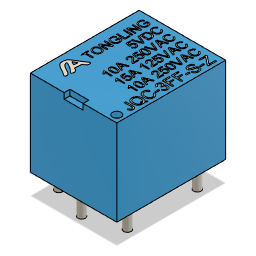
5v Cube Relay (Autodesk Fusion 360 design; units mm, degrees)
Autodesk Fusion 360 part; units mm, degrees
(part 1 of 2)
sketch "Sketch1" plane through (0, 0, 0) normal (0, 1, 0) x (1, 0, 0)
  line L0 (0, 0) -> (26, 0)
  line L1 (26, 0) -> (26, 33.5)
  line L2 (26, 33.5) -> (0, 33.5)
  line L3 (0, 33.5) -> (0, 0)
  line L4 (2.275, 33.5) -> (2.275, 0) construction
  circle A0 centre (2.275, 31.325) radius 1.475
  circle A1 centre (2.275, 2.375) radius 1.475
  line L5 (13, 33.5) -> (13, 0) construction
  circle A2 centre (23.725, 31.325) radius 1.475
  circle A3 centre (23.725, 2.375) radius 1.475
  dimension "d1" = 26
  dimension "d2" = 33.5
  dimension "d3" = 2.95
  dimension "d4" = 0.75
  dimension "d5" = 0.7
  dimension "d7" = 2.225
  dimension "d9" = 26
  dimension "d10" = 0.9
  dimension "d11" = 18.5
  constraint horizontal L0
  constraint vertical L1
  constraint horizontal L2
  constraint vertical L3
  constraint coincident L0.start L3.end
  constraint coincident L2 L4.start
  constraint coincident L0 L4.end
  constraint perpendicular L0 L4
  constraint coincident L4 A0.centre
  constraint coincident L4 A1.centre
  constraint equal A0 A1
  constraint midpoint L2 L5.start
  constraint midpoint L0 L5.end
  constraint symmetric A0 L5 A2
  constraint symmetric A1 L5 A3
  measures "d1" distance of L0.start L0.end
  measures "d2" distance of L0.start L2.end
  measures "d3" diameter of A0
  measures "d5" distance of L2 A0
  measures "d9" distance of A0 A1
  measures "d10" distance of L0 A1
  measures "d11" distance of A1 A3
sketch "Sketch2" plane through (0, 1.55, 0) normal (0, 1, 0) x (-1, 0, 0)
  circle A0 centre (-2.275, -2.375) radius 1.475
  circle A1 centre (-23.725, -2.375) radius 1.475
  circle A2 centre (-23.725, -31.325) radius 1.475
  circle A3 centre (-2.275, -31.325) radius 1.475
  line L0 (0, -33.5) -> (0, 0)
  line L1 (0, 0) -> (-26, 0)
  line L2 (-26, 0) -> (-26, -33.5)
  line L3 (-26, -33.5) -> (0, -33.5)
  line L4 (-5.9, -23.5) -> (-21, -23.5)
  line L5 (-21, -23.5) -> (-21, -4.5)
  line L6 (-21, -4.5) -> (-5.9, -4.5)
  line L7 (-5.9, -4.5) -> (-5.9, -23.5)
  dimension "d14" = 15.1
  dimension "d15" = 19
  dimension "d16" = 10
  dimension "d17" = 5
  dimension "d18" = 5.9
  dimension "d19" = 4.75
  constraint horizontal L4
  constraint vertical L5
  constraint horizontal L6
  constraint vertical L7
  measures "d14" distance of L4.start L4.end
  measures "d15" distance of L4.start L6.end
  measures "d16" distance of L3 L4
  measures "d17" distance of L2 L5
  measures "d18" distance of L0 L7
extrude "Extrude2" add sketch "Sketch2" along normal blind 15 contours L4 L5 L6 L7 makes body 1
sketch "Sketch3" plane through (0, 16.55, 0) normal (0, 1, 0) x (-1, 0, 0)
  line L0 (-5.9, -4.5) -> (-21, -4.5)
  line L1 (-21, -4.5) -> (-21, -23.5)
  line L2 (-21, -23.5) -> (-5.9, -23.5)
  line L3 (-5.9, -23.5) -> (-5.9, -4.5)
  circle A0 centre (-19.75, -5.75) radius 0.75
  line L4 (-15.1, -5.5) -> (-11.8, -5.5)
  line L5 (-11.8, -5.5) -> (-11.8, -3.5)
  line L6 (-11.8, -3.5) -> (-15.1, -3.5)
  line L7 (-15.1, -3.5) -> (-15.1, -5.5)
  line L8 (-15.1, -5.5) -> (-11.8, -3.5) construction
  line L9 (-11.8, -5.5) -> (-15.1, -3.5) construction
  point P0 (-13.45, -4.5)
  dimension "d22" = 1.5
  dimension "d23" = 0.5
  dimension "d24" = 0.5
  dimension "d25" = 1
  dimension "d26" = 3.3
  constraint horizontal L4
  constraint perpendicular L4 L5
  constraint parallel L4 L6
  constraint parallel L5 L7
  constraint coincident L8 P0
  constraint coincident L9 P0
  constraint midpoint L0 P0
  measures "d22" diameter of A0
  measures "d23" distance of L0 A0
  measures "d24" distance of L1 A0
  measures "d25" distance of L0 L4
  measures "d26" distance of L5.end L6.end
extrude "Extrude3" cut sketch "Sketch3" against normal blind 1 contours L0 L4 L5 L7 | L0 L5 L6 L7 | A0 bodies 1
sketch "Sketch4" plane through (0, 16.55, 0) normal (0, 1, 0) x (-1, 0, 0)
  line L0 (-11.8, -4.5) -> (-11.8, -5.5)
  line L1 (-11.8, -5.5) -> (-15.1, -5.5)
  line L2 (-15.1, -5.5) -> (-15.1, -4.5)
  line L3 (-15.1, -4.5) -> (-21, -4.5)
  line L4 (-21, -4.5) -> (-21, -23.5)
  line L5 (-21, -23.5) -> (-5.9, -23.5)
  line L6 (-5.9, -23.5) -> (-5.9, -4.5)
  line L7 (-5.9, -4.5) -> (-11.8, -4.5)
  circle A0 centre (-19.75, -5.75) radius 0.75
sketch "Sketch5" plane through (0, 1.55, 0) normal (0, 1, 0) x (-1, 0, 0)
  circle A0 centre (-2.275, -2.375) radius 1.475
  circle A1 centre (-23.725, -2.375) radius 1.475
  circle A2 centre (-23.725, -31.325) radius 1.475
  circle A3 centre (-2.275, -31.325) radius 1.475
  line L0 (0, -33.5) -> (0, 0)
  line L1 (0, 0) -> (-26, 0)
  line L2 (-26, 0) -> (-26, -33.5)
  line L3 (-26, -33.5) -> (0, -33.5)
  line L4 (-13.38, -3.54) -> (-21, -3.54)
  line L5 (-21, -3.54) -> (-21, -1)
  line L6 (-21, -1) -> (-13.38, -1)
  line L7 (-13.38, -1) -> (-13.38, -3.54)
  line L8 (-15.92, -3.54) -> (-15.92, -1) construction
  line L9 (-18.46, -3.54) -> (-18.46, -1) construction
  line L10 (-15.412, -3.54) -> (-15.92, -3.032)
  line L11 (-17.19, -3.54) -> (-17.19, -1) construction
  line L12 (-13.38, -2.27) -> (-17.19, -2.27) construction
  line L13 (-14.65, -3.54) -> (-14.65, -1) construction
  line L14 (-13.38, -3.032) -> (-13.888, -3.54)
  line L15 (-16.428, -3.54) -> (-15.92, -3.032)
  line L16 (-13.38, -1.508) -> (-13.888, -1)
  line L17 (-15.412, -1) -> (-15.92, -1.508)
  line L18 (-16.428, -1) -> (-15.92, -1.508)
  line L19 (-21, -3.032) -> (-20.492, -3.54)
  line L20 (-21, -1.508) -> (-20.492, -1)
  line L21 (-18.968, -1) -> (-18.46, -1.508)
  line L22 (-18.968, -3.54) -> (-18.46, -3.032)
  line L23 (-17.952, -3.54) -> (-18.46, -3.032)
  line L24 (-17.952, -1) -> (-18.46, -1.508)
  dimension "d29" = 7.62
  dimension "d30" = 2.54
  dimension "d31" = 5
  dimension "d32" = 1
  dimension "d33" = 2.54
  dimension "d34" = 2.54
  dimension "d35" = 45
  dimension "d36" = 0.508
  dimension "d37" = 1.27
  dimension "d38" = 45
  constraint horizontal L4
  constraint vertical L5
  constraint horizontal L6
  constraint vertical L7
  constraint coincident L4 L8.start
  constraint coincident L6 L8.end
  constraint perpendicular L6 L8
  constraint coincident L4 L9.start
  constraint coincident L6 L9.end
  constraint perpendicular L6 L9
  constraint coincident L4 L10.start
  constraint coincident L8 L10.end
  constraint midpoint L4 L11.start
  constraint midpoint L6 L11.end
  constraint midpoint L7 L12.start
  constraint midpoint L11 L12.end
  constraint coincident L4 L13.start
  constraint coincident L6 L13.end
  constraint perpendicular L6 L13
  constraint coincident L7 L14.start
  constraint coincident L4 L14.end
  constraint horizontal L10.end L14.start
  constraint symmetric L8 L10.start L15.start
  constraint symmetric L8 L10.end L15.end
  constraint symmetric L10.start L12 L17.start
  constraint symmetric L10.end L12 L17.end
  constraint symmetric L12 L14.start L16.start
  constraint symmetric L12 L14.end L16.end
  constraint symmetric L12 L15.start L18.start
  constraint symmetric L12 L10.end L17.end
  constraint symmetric L10.start L11 L22.start
  constraint symmetric L10.end L11 L22.end
  constraint symmetric L11 L14.start L19.start
  constraint symmetric L11 L14.end L19.end
  constraint symmetric L11 L15.start L23.start
  constraint symmetric L11 L10.end L22.end
  constraint symmetric L11 L16.start L20.start
  constraint symmetric L11 L16.end L20.end
  constraint symmetric L11 L17.start L21.start
  constraint symmetric L11 L17.end L21.end
  constraint symmetric L11 L18.start L24.start
  measures "d29" distance of L4.start L4.end
  measures "d30" distance of L4.start L6.end
  measures "d31" distance of L2 L5
  measures "d32" distance of L1 L6
  measures "d33" distance of L8 L9
  measures "d34" distance of L7 L8
  measures "d35" angle of L8 L10
  measures "d36" distance of L8.start L10.end
  measures "d37" distance of L7 L13
  measures "d38" angle of L7 L14
sketch "Sketch8" plane through (0, 4.09, 0) normal (0, 1, 0) x (-1, 0, 0)
  line L0 (-16.428, -1) -> (-17.952, -1)
  line L1 (-17.952, -1) -> (-18.46, -1.508)
  line L2 (-18.46, -1.508) -> (-18.968, -1)
  line L3 (-18.968, -1) -> (-20.492, -1)
  line L4 (-20.492, -1) -> (-21, -1.508)
  line L5 (-21, -1.508) -> (-21, -3.032)
  line L6 (-21, -3.032) -> (-20.492, -3.54)
  line L7 (-20.492, -3.54) -> (-18.968, -3.54)
  line L8 (-18.968, -3.54) -> (-18.46, -3.032)
  line L9 (-18.46, -3.032) -> (-17.952, -3.54)
  line L10 (-17.952, -3.54) -> (-16.428, -3.54)
  line L11 (-16.428, -3.54) -> (-15.92, -3.032)
  line L12 (-15.92, -3.032) -> (-15.412, -3.54)
  line L13 (-15.412, -3.54) -> (-13.888, -3.54)
  line L14 (-13.888, -3.54) -> (-13.38, -3.032)
  line L15 (-13.38, -3.032) -> (-13.38, -1.508)
  line L16 (-13.38, -1.508) -> (-13.888, -1)
  line L17 (-13.888, -1) -> (-15.412, -1)
  line L18 (-15.412, -1) -> (-15.92, -1.508)
  line L19 (-15.92, -1.508) -> (-16.428, -1)
  line L20 (-15.92, -3.032) -> (-15.92, -1.508) construction
  line L21 (-17.19, -3.54) -> (-17.19, -1) construction
  line L22 (-15.87, -3.54) -> (-15.87, -1)
  line L23 (-15.87, -1) -> (-15.97, -1)
  line L24 (-15.97, -1) -> (-15.97, -3.54)
  line L25 (-15.97, -3.54) -> (-15.87, -3.54)
  line L26 (-18.51, -3.54) -> (-18.51, -1)
  line L27 (-18.41, -1) -> (-18.41, -3.54)
  line L28 (-18.41, -3.54) -> (-18.51, -3.54)
  line L29 (-18.51, -1) -> (-18.41, -1)
  dimension "d55" = 0.1
  dimension "d56" = 0.05
  constraint coincident L11.end L12.start
  constraint coincident L18.end L19.start
  constraint midpoint L10 L21.start
  constraint midpoint L0 L21.end
  constraint vertical L22
  constraint perpendicular L22 L23
  constraint perpendicular L23 L24
  constraint perpendicular L22 L25
  constraint collinear L10 L25
  constraint collinear L0 L23
  constraint symmetric L21 L22.start L26.start
  constraint symmetric L21 L22.end L26.end
  constraint symmetric L21 L23.end L27.start
  constraint symmetric L21 L24.end L27.end
  measures "d55" distance of L22.start L24.end
  measures "d56" distance of L20 L24
sketch "Negative Pin" plane through (13.38, 0, 0) normal (-1, 0, 0) x (0, 0, 1)
  line L0 (-3.032, 1.55) -> (-1.508, 1.55)
  line L1 (-1.508, 1.55) -> (-1.508, 4.09)
  line L2 (-1.508, 4.09) -> (-3.032, 4.09)
  line L3 (-3.032, 4.09) -> (-3.032, 1.55)
  line L4 (-3.032, 1.55) -> (-1.508, 1.55)
  line L5 (-1.508, 1.55) -> (-1.508, 1.8)
  line L6 (-1.508, 1.8) -> (-3.032, 1.8)
  line L7 (-3.032, 1.8) -> (-3.032, 1.55)
  dimension "d59" = 0.25
  constraint horizontal L4
  constraint vertical L5
  constraint horizontal L6
  constraint vertical L7
  constraint coincident L1 L5.end
  constraint coincident L0.start L3.end
  measures "d59" distance of L0.start L6.end
ref_plane "WorkPlane1" through (13, 0.775, 5) normal (0, 0, 1) x (1, 0, 0)
sketch "Sketch10" plane through (13, 0.775, 5) normal (0, 0, 1) x (1, 0, 0)
  line L0 (6.73, -0.775) -> (6.73, 5.225) construction
  line L1 (-13, -0.775) -> (13, -0.775) construction
  line L2 (5.968, 0.775) -> (5.968, 3.315) construction
  line L3 (7.492, 0.775) -> (7.492, 3.315) construction
  line L4 (6.48, 5.225) -> (6.98, 5.225)
  line L5 (6.98, 5.225) -> (6.98, 4.725)
  line L6 (6.98, 4.725) -> (6.48, 4.725)
  line L7 (6.48, 4.725) -> (6.48, 5.225)
  dimension "d63" = 6
  dimension "d64" = 0.5
  dimension "d65" = 0.5
  constraint vertical L0
  constraint coincident L0.start L1
  constraint symmetric L0 L2 L3
  constraint horizontal L4
  constraint vertical L5
  constraint horizontal L6
  constraint vertical L7
  constraint coincident L0.end L4
  constraint midpoint L0.end L4
  measures "d63" distance of L0.start L0.end
  measures "d64" distance of L4.start L4.end
  measures "d65" distance of L4.start L6.end
ref_plane "WorkPlane2" through (19.73, 2.82, -2.27) normal (1, 0, 0) x (0, 0, -1)
sketch "Sketch11" plane through (19.73, 2.945, -2.27) normal (1, 0, 0) x (0, 0, -1)
  line L0 (-7.27, 2.805) -> (-0.25, 2.805)
  line L1 (0, 2.555) -> (0, -4.195)
  line L2 (-7.27, 3.055) -> (-7.27, 2.555)
  line L3 (-2.27, -2.945) -> (31.23, -2.945)
  arc A0 (0, 2.555) -> (-0.25, 2.805) centre (-0.25, 2.555) ccw
  line L4 (-0.762, -1.145) -> (-0.762, 1.145)
  line L5 (0.762, -1.145) -> (0.762, 1.145)
  dimension "d67" = 1.25
  dimension "d68" = 0.25
  constraint horizontal L0
  constraint perpendicular L0 L1
  constraint midpoint L0.start L2
  constraint tangent L0 A0
  constraint tangent L1 A0
  measures "d67" distance of L1.end L3
  measures "d68" radius of A0
sketch "Sketch12" plane through (5.9, 0, 0) normal (-1, 0, 0) x (0, 0, 1)
  line L0 (-23.5, 1.55) -> (-4.5, 1.55)
  line L1 (-4.5, 1.55) -> (-4.5, 16.55)
  line L2 (-4.5, 16.55) -> (-23.5, 16.55)
  line L3 (-23.5, 16.55) -> (-23.5, 1.55)
  line L4 (-31.2, 1.55) -> (-23.6, 1.55)
  line L5 (-23.6, 1.55) -> (-23.6, 8.05)
  line L6 (-31.2, 8.05) -> (-31.2, 1.55)
  line L7 (-33.5, 1.55) -> (0, 1.55)
  line L8 (-30.4, 11.55) -> (-25.4, 11.55)
  line L9 (-30.4, 11.55) -> (-31.2, 8.05)
  line L10 (-25.4, 11.55) -> (-23.6, 8.05)
  line L11 (-31.2, 8.05) -> (-23.6, 8.05) construction
  dimension "d83" = 7.6
  dimension "d84" = 6.5
  dimension "d85" = 0.1
  dimension "d86" = 5
  dimension "d89" = 1.8
  dimension "d90" = 3.5
  constraint horizontal L4
  constraint vertical L5
  constraint vertical L6
  constraint collinear L4 L7
  constraint horizontal L8
  constraint horizontal L5.end L6.start
  measures "d83" distance of L4.start L4.end
  measures "d84" distance of L4.start L6.start
  measures "d85" distance of L3 L5
  measures "d86" distance of L8.start L8.end
  measures "d89" horizontal distance of L5.end L8.end
  measures "d90" distance of L6.start L8
sketch "Sketch13" plane through (0, 0, -31.2) normal (0, 0, -1) x (-1, 0, 0)
  line L0 (-5.9, 1.55) -> (-5.9, 8.05)
  line L1 (-5.9, 8.05) -> (-20.9, 8.05)
  line L2 (-20.9, 8.05) -> (-20.9, 1.55)
  line L3 (-20.9, 1.55) -> (-5.9, 1.55)
  line L4 (-20.4, 7.55) -> (-16.4, 7.55)
  line L5 (-16.4, 7.55) -> (-16.4, 2.55)
  line L6 (-16.4, 2.55) -> (-20.4, 2.55)
  line L7 (-20.4, 2.55) -> (-20.4, 7.55)
  dimension "d93" = 4
  dimension "d94" = 5
  dimension "d95" = 0.5
  dimension "d97" = 1
  constraint horizontal L4
  constraint vertical L5
  constraint horizontal L6
  constraint vertical L7
  measures "d93" distance of L4.start L4.end
  measures "d94" distance of L4.start L6.end
  measures "d95" distance of L2 L7
  measures "d97" distance of L3 L6
pattern_linear "R-Pattern2" [no effect]
sketch "Sketch14" plane through (0, 11.55, 0) normal (0, 1, 0) x (-1, 0, 0)
  line L0 (-5.9, -30.4) -> (-5.9, -25.4)
  line L1 (-5.9, -25.4) -> (-20.9, -25.4)
  line L2 (-20.9, -25.4) -> (-20.9, -30.4)
  line L3 (-20.9, -30.4) -> (-5.9, -30.4)
  line L4 (-20.9, -28.1) -> (-5.9, -28.1) construction
  line L5 (-5.9, -23.6) -> (-20.9, -23.6) construction
  circle A0 centre (-18.4, -28.1) radius 2
  dimension "d104" = 4.5
  dimension "d105" = 4
  dimension "d106" = 0.5
  constraint coincident L2 L4.start
  constraint coincident L0 L4.end
  constraint perpendicular L0 L4
  constraint coincident L4 A0.centre
  measures "d104" distance of L4 L5
  measures "d105" diameter of A0
  measures "d106" distance of L2 A0
pattern_linear "R-Pattern3" [no effect]
sketch "Sketch15" plane through (0, 2.55, 0) normal (0, 1, 0) x (-1, 0, 0)
  line L0 (-20.4, -31.2) -> (-16.4, -31.2)
  line L1 (-16.4, -31.2) -> (-16.4, -25.4)
  line L2 (-16.4, -25.4) -> (-20.4, -25.4)
  line L3 (-20.4, -25.4) -> (-20.4, -31.2)
  line L4 (-5.9, -23.6) -> (-20.9, -23.6)
  line L5 (-17.9, -28.1) -> (-17.9, -31.2)
  line L6 (-18.9, -31.2) -> (-18.9, -28.1)
  arc A0 (-17.9, -28.1) -> (-18.9, -28.1) centre (-18.4, -28.1) ccw
  line L7 (-17.9, -31.2) -> (-18.9, -31.2)
  dimension "d113" = 1
  dimension "d114" = 4.5
  dimension "d115" = 2
  constraint coincident L0 L5.end
  constraint perpendicular L0 L5
  constraint coincident L0 L6.start
  constraint vertical L6
  constraint tangent L5 A0
  constraint tangent L6 A0
  measures "d113" diameter of A0
  measures "d114" distance of A0.centre L4
  measures "d115" distance of L3 A0.centre
pattern_linear "R-Pattern4" [no effect]
sketch "Sketch16" plane through (0, 0, -25.4) normal (0, 0, -1) x (-1, 0, 0)
  line L0 (-20.4, 2.55) -> (-16.4, 2.55)
  line L1 (-16.4, 2.55) -> (-16.4, 7.55)
  line L2 (-16.4, 7.55) -> (-20.4, 7.55)
  line L3 (-20.4, 7.55) -> (-20.4, 2.55)
  line L4 (-18.4, 7.55) -> (-18.4, 2.55) construction
  circle A0 centre (-18.4, 4.45) radius 1.4
  line L5 (-18.9, 1.55) -> (-20.9, 1.55)
  dimension "d122" = 2.8
  dimension "d123" = 2.9
  constraint midpoint L2 L4.start
  constraint midpoint L0 L4.end
  constraint coincident L4 A0.centre
  measures "d122" diameter of A0
  measures "d123" distance of A0.centre L5
ref_plane "WorkPlane3" through (13.4, -2.2, -27.4) normal (0, -1, 0) x (0, 0, -1)
sketch "Sketch17" plane through (13.4, -2.2, -27.4) normal (0, -1, 0) x (1, 0, 0)
  circle A0 centre (5, -0.7) radius 0.5
  arc A1 (5.5, -0.7) -> (4.5, -0.7) centre (5, -0.7) ccw
  dimension "d127" = 1
  constraint concentric A0 A1
  measures "d127" diameter of A0
combine "Combine3" [no effect]
sketch "Sketch18" plane through (0, 7.55, 0) normal (0, 1, 0) x (-1, 0, 0)
  line L0 (-16.4, -25.4) -> (-20.4, -25.4)
  line L1 (-20.4, -25.4) -> (-20.4, -30.1)
  line L2 (-20.4, -30.1) -> (-16.4, -30.1)
  line L3 (-16.4, -30.1) -> (-16.4, -25.4)
  circle A0 centre (-18.4, -28.1) radius 0.84
  circle A1 centre (-18.4, -28.1) radius 2
  dimension "d130" = 1.68
  constraint concentric A0 A1
  measures "d130" diameter of A0
ref_plane "WorkPlane4" through (13.4, 8.55, -27.9) normal (0, 1, 0) x (0, 0, 1)
sketch "Sketch21" plane through (13.4, 8.55, -27.9) normal (0, 1, 0) x (1, 0, 0)
  circle A0 centre (5, 0.2) radius 0.84
sketch "Sketch22" plane through (0, 8.55, 0) normal (0, 1, 0) x (-1, 0, 0)
  circle A0 centre (-18.4, -28.1) radius 0.84
  circle A1 centre (-18.4, -28.1) radius 2
combine "Combine4" [no effect]
sketch "Sketch23" plane through (0, 10.55, 0) normal (0, 1, 0) x (-1, 0, 0)
  circle A0 centre (-18.4, -28.1) radius 2
  line L0 (-18.4, -28.1) -> (-20.4, -28.1) construction
  line L1 (-20.3645, -28.475) -> (-16.4355, -28.475)
  line L2 (-16.4355, -27.725) -> (-20.3645, -27.725)
  arc A1 (-16.4355, -28.475) -> (-16.4355, -27.725) centre (-18.4, -28.1) ccw
  arc A2 (-20.3645, -27.725) -> (-20.3645, -28.475) centre (-18.4, -28.1) ccw
  dimension "d138" = 0.75
  dimension "d139" = 0.375
  dimension "d140" = 2
  dimension "d141" = 2
  constraint coincident A0.centre L0.start
  constraint coincident A0 L0.end
  constraint horizontal L0
  constraint horizontal L1
  constraint horizontal L2
  constraint coincident A0 L2.start
  constraint coincident A0 L1.start
  constraint concentric A1 A2
  measures "d138" distance of L1 L2
  measures "d139" distance of L0 L2
  measures "d140" radius of A1
  measures "d141" radius of A2
combine "Combine7" [no effect]
combine "Combine8" [no effect]
sketch "Sketch24" plane through (0, 0, 0) normal (0, -1, 0) x (1, 0, 0)
  circle A0 centre (8.4, -28.1) radius 0.5
  circle A1 centre (13.4, -28.1) radius 0.5
  circle A2 centre (18.4, -28.1) radius 0.5
  line L0 (19.98, -2.52) -> (19.48, -2.52)
  line L1 (19.48, -2.52) -> (19.48, -2.02)
  line L2 (19.48, -2.02) -> (19.98, -2.02)
  line L3 (19.98, -2.02) -> (19.98, -2.52)
  line L4 (17.44, -2.52) -> (16.94, -2.52)
  line L5 (16.94, -2.52) -> (16.94, -2.02)
  line L6 (16.94, -2.02) -> (17.44, -2.02)
  line L7 (17.44, -2.02) -> (17.44, -2.52)
  line L8 (14.9, -2.52) -> (14.4, -2.52)
  line L9 (14.4, -2.52) -> (14.4, -2.02)
  line L10 (14.4, -2.02) -> (14.9, -2.02)
  line L11 (14.9, -2.02) -> (14.9, -2.52)
  circle A3 centre (2.275, -2.375) radius 1.475
  circle A4 centre (23.725, -2.375) radius 1.475
  circle A5 centre (23.725, -31.325) radius 1.475
  circle A6 centre (2.275, -31.325) radius 1.475
  line L12 (0, 0) -> (0, -33.5)
  line L13 (0, -33.5) -> (26, -33.5)
  line L14 (26, -33.5) -> (26, 0)
  line L15 (26, 0) -> (0, 0)
  circle A7 centre (19.45, -7.9) radius 0.65
  line L16 (7.45, -20.1) -> (19.45, -20.1) construction
  circle A8 centre (7.45, -20.1) radius 0.65
  circle A9 centre (19.45, -20.1) radius 0.65
  circle A10 centre (7.45, -7.9) radius 0.65
  line L17 (7.45, -7.9) -> (19.45, -7.9) construction
  line L18 (21, -4.5) -> (5.9, -4.5) construction
  line L19 (5.9, -4.5) -> (5.9, -23.5) construction
  line L20 (5.9, -23.5) -> (21, -23.5) construction
  line L21 (21, -23.5) -> (21, -4.5) construction
  line L22 (13.45, -23.5) -> (13.45, -4.5) construction
  circle A11 centre (13.45, -5.9) radius 0.65
  dimension "d148" = 1.3
  dimension "d151" = 12
  dimension "d152" = 12
  dimension "d153" = 12.2
  dimension "d157" = 3.4
  dimension "d158" = 2
  constraint horizontal L16
  constraint coincident L16.start A8.centre
  constraint coincident L16.end A9.centre
  constraint coincident A10.centre L17.start
  constraint coincident A7.centre L17.end
  constraint equal A9 A10
  constraint equal A7 A10
  constraint midpoint L20 L22.start
  constraint midpoint L18 L22.end
  constraint symmetric L16.start L16.end L22
  constraint symmetric A7.centre A10.centre L22
  constraint coincident L22 A11.centre
  constraint equal A7 A11
  measures "d148" diameter of A7
  measures "d151" distance of A10.centre A7.centre
  measures "d152" distance of L16.start L16.end
  measures "d153" distance of A7.centre L16.end
  measures "d157" distance of L16.end L20
  measures "d158" distance of L17 A11.centre
extrude "Extrude19" add sketch "Sketch24" along normal blind 2 and the other way up to surface (1.55 mm away) separate body contours A7 | A8 | A9 | A10 | A11 makes body 2 at (19.243, -1.3333, -7.2838) makes body 3 at (19.243, -1.3333, -19.4838) makes body 4 at (12.9961, -1.3333, -6.3653) makes body 5 at (8.0992, -1.3333, -20.1324) makes body 6 at (8.0992, -1.3333, -7.9324)
sketch "Sketch26" plane through (0, 16.55, 0) normal (0, 1, 0) x (-1, 0, 0)
  line L0 (-11.8, -4.5) -> (-11.8, -5.5)
  line L1 (-11.8, -5.5) -> (-15.1, -5.5)
  line L2 (-15.1, -5.5) -> (-15.1, -4.5)
  line L3 (-15.1, -4.5) -> (-21, -4.5)
  line L4 (-21, -4.5) -> (-21, -23.5)
  line L5 (-21, -23.5) -> (-5.9, -23.5)
  line L6 (-5.9, -23.5) -> (-5.9, -4.5)
  line L7 (-5.9, -4.5) -> (-11.8, -4.5)
  circle A0 centre (-19.75, -5.75) radius 0.75
  line L8 (-8.4415, -9.5193) -> (-8.5, -10.25)
  line L9 (-8.5, -10.25) -> (-7.8, -9.85)
  line L10 (-7.8, -9.85) -> (-8.4415, -9.5193)
  line L11 (-9, -9.1) -> (-9.1, -10.35)
  line L12 (-9.7, -10.8) -> (-9.7, -11.25)
  line L13 (-9.65, -11.3) -> (-9.4, -11.3)
  line L14 (-9.1853, -7.053) -> (-9.3987, -7.053)
  line L15 (-9.4487, -7.103) -> (-9.4487, -7.4)
  spline S0 degree 5 poles (-9.1853, -7.053) (-9.0822, -7.1318) (-8.8783, -7.2798) (-8.5798, -7.4735) (-8.1986, -7.6824) (-7.7638, -7.9025) (-7.3929, -8.1291) (-7.1114, -8.3991) (-6.9553, -8.7258) (-6.952, -9.0743) (-7.0055, -9.3778) (-7.04, -9.5928) (-7.0826, -9.7454) (-7.3804, -9.9863) (-7.9114, -10.3237) (-8.5564, -10.7138) (-9.017, -11.0032) (-9.2583, -11.174) (-9.3623, -11.2623) (-9.4, -11.3) knots 0 0 0 0 0 0 0.066667 0.133333 0.2 0.266667 0.333333 0.4 0.466667 0.533333 0.6 0.666667 0.733333 0.8 0.866667 0.933333 1 1 1 1 1 1
  line L16 (-9.7707, -6.6059) -> (-8.6, -7.5)
  line L17 (-7.2894, -8.1164) -> (-6.8512, -8.9402)
  line L18 (-6.9688, -9.4269) -> (-7.17, -9.8796)
  line L19 (-9.2, -11.1) -> (-9.6, -11.5)
  spline S1 degree 5 poles (-9.4487, -7.4) (-9.446, -7.4214) (-9.4369, -7.4643) (-9.4123, -7.5287) (-9.3574, -7.615) (-9.2517, -7.7235) (-9.1097, -7.8329) (-8.9344, -7.9436) (-8.7324, -8.0561) (-8.5144, -8.1715) (-8.2929, -8.2908) (-8.0811, -8.415) (-7.8911, -8.5451) (-7.733, -8.6818) (-7.6123, -8.8255) (-7.5314, -8.9763) (-7.499, -9.1024) (-7.4926, -9.2) (-7.4962, -9.2664) (-7.5, -9.3) knots 0 0 0 0 0 0 0.066667 0.133333 0.2 0.266667 0.333333 0.4 0.466667 0.533333 0.6 0.666667 0.733333 0.8 0.866667 0.933333 1 1 1 1 1 1
  spline S2 degree 5 poles (-7.5, -9.3) (-7.5453, -9.28) (-7.6351, -9.2397) (-7.7677, -9.1777) (-7.9404, -9.0923) (-8.1488, -8.9806) (-8.3491, -8.8635) (-8.5405, -8.7404) (-8.7227, -8.6112) (-8.8959, -8.4759) (-9.0608, -8.3352) (-9.1866, -8.2185) (-9.2778, -8.1288) (-9.3372, -8.0681) (-9.3665, -8.0375) knots 0 0 0 0 0 0 0.1 0.2 0.3 0.4 0.5 0.6 0.7 0.8 0.9 1 1 1 1 1 1
  spline S3 degree 5 poles (-9.3665, -8.0375) (-9.3865, -8.0328) (-9.4244, -8.0261) (-9.4743, -8.024) (-9.5273, -8.0375) (-9.5711, -8.0811) (-9.5952, -8.1493) (-9.6052, -8.2368) (-9.6135, -8.3325) (-9.6222, -8.4296) (-9.627, -8.5246) (-9.6199, -8.6162) (-9.5923, -8.7043) (-9.5374, -8.7891) (-9.4523, -8.871) (-9.3355, -8.9502) (-9.2169, -9.0114) (-9.1138, -9.0561) (-9.039, -9.0855) (-9, -9.1) knots 0 0 0 0 0 0 0.066667 0.133333 0.2 0.266667 0.333333 0.4 0.466667 0.533333 0.6 0.666667 0.733333 0.8 0.866667 0.933333 1 1 1 1 1 1
  line L20 (-9.5778, -8.0418) -> (-9.6222, -8.3582)
  arc A1 (-9.3987, -7.053) -> (-9.4487, -7.103) centre (-9.3987, -7.103) ccw
  arc A2 (-9.7, -11.25) -> (-9.65, -11.3) centre (-9.65, -11.25) ccw
  spline S4 degree 5 poles (-9.1, -10.35) (-9.1212, -10.3601) (-9.1639, -10.3811) (-9.2289, -10.4154) (-9.3178, -10.4671) (-9.434, -10.5464) (-9.5337, -10.629) (-9.6143, -10.7072) (-9.6709, -10.7677) (-9.7, -10.8) knots 0 0 0 0 0 0 0.2 0.4 0.6 0.8 1 1 1 1 1 1
  line L21 (-9.6266, -10.7183) -> (-9.7734, -10.8817)
  line L22 (-9.05, -11.6493) -> (-9.05, -22.6569) construction
  line L23 (-11.25, -22.6569) -> (-11.25, -16.691) construction
  line L24 (-5.9, -22.6569) -> (-21, -22.6569) construction
  line L25 (-13.45, -10.5) -> (-13.45, -22.6569) construction
  line L26 (-15.65, -10.5) -> (-15.65, -22.6569) construction
  line L27 (-17.85, -10.5) -> (-17.85, -22.6569) construction
  line L28 (-20.35, -7.4097) -> (-20.35, -22.6569) construction
  point P0 (-7.0703, -8.5283)
  point P1 (-7.0694, -9.6533)
  point P2 (-9, -7.9)
  point P3 (-7.8722, -8.5678)
  point P4 (-8.5514, -8.7299)
  point P5 (-9.6, -8.2)
  point P6 (-9.6031, -8.6598)
  dimension "d163" = 0.05
  dimension "d164" = 0.05
  dimension "d167" = 2.2
  dimension "d169" = 2.2
  dimension "d170" = 3.15
  dimension "d171" = 2.2
  dimension "d172" = 2.2
  dimension "d173" = 2.5
  text T0 "TONGLING" font "Arial" height 1.5 align left spacing 1 along the path L22 letters at x, y, angle (-7.153, -11.6493, -90) (-7.153, -12.9293, -90) (-7.153, -14.5592, -90) (-7.153, -16.0725, -90) (-7.153, -17.7025, -90) (-7.153, -18.8679, -90) (-7.153, -19.4501, -90) (-7.153, -20.9634, -90)
  text T1 "5VDC" font "Arial" height 1.5 align left spacing 1 along the path L23 letters at x, y, angle (-9.353, -17.0672, -90) (-9.353, -18.2326, -90) (-9.353, -19.6303, -90) (-9.353, -21.1436, -90)
  text T2 "10A 250VAC" font "Arial" height 1.5 align left spacing 1 along the path L25 letters at x, y, angle (-11.553, -10.5, -90) (-11.553, -11.6654, -90) (-11.553, -12.8308, -90) (-11.553, -14.2347, -90) (-11.553, -14.8168, -90) (-11.553, -15.9823, -90) (-11.553, -17.1477, -90) (-11.553, -18.3131, -90) (-11.553, -19.7108, -90) (-11.553, -21.1146, -90)
  text T3 "15A 125VAC" font "Arial" height 1.5 align left spacing 1 along the path L26 letters at x, y, angle (-13.753, -10.5, -90) (-13.753, -11.6654, -90) (-13.753, -12.8308, -90) (-13.753, -14.2347, -90) (-13.753, -14.8168, -90) (-13.753, -15.9823, -90) (-13.753, -17.1477, -90) (-13.753, -18.3131, -90) (-13.753, -19.7108, -90) (-13.753, -21.1146, -90)
  text T4 "10A 250VAC" font "Arial" height 1.5 align left spacing 1 along the path L27 letters at x, y, angle (-15.953, -10.5, -90) (-15.953, -11.6654, -90) (-15.953, -12.8308, -90) (-15.953, -14.2347, -90) (-15.953, -14.8168, -90) (-15.953, -15.9823, -90) (-15.953, -17.1477, -90) (-15.953, -18.3131, -90) (-15.953, -19.7108, -90) (-15.953, -21.1146, -90)
  text T5 "JQC-3FF-S-Z" font "Arial" height 1.8 align left spacing 1 along the path L28 letters at x, y, angle (-18.0736, -7.4097, -90) (-18.0736, -8.667, -90) (-18.0736, -10.623, -90) (-18.0736, -12.4389, -90) (-18.0736, -13.2763, -90) (-18.0736, -14.6748, -90) (-18.0736, -16.2108, -90) (-18.0736, -17.7468, -90) (-18.0736, -18.5842, -90) (-18.0736, -20.2614, -90) (-18.0736, -21.0988, -90)
  constraint parallel L8 L11
  constraint vertical L12
  constraint perpendicular L12 L13
  constraint horizontal L14
  constraint perpendicular L14 L15
  constraint midpoint L14.start L16
  constraint midpoint P0 L17
  constraint midpoint P1 L18
  constraint midpoint L13.end L19
  constraint midpoint P5 L20
  constraint tangent L14 A1
  constraint tangent L15 A1
  constraint tangent L12 A2
  constraint tangent L13 A2
  constraint midpoint L12.start L21
  constraint vertical L22
  constraint perpendicular L5 L23
  constraint coincident L6 L24.start
  constraint coincident L4 L24.end
  constraint perpendicular L4 L24
  constraint coincident L22.end L24
  constraint coincident L23.start L24
  constraint midpoint L24 L25.end
  constraint vertical L25
  constraint coincident L24 L26.end
  constraint perpendicular L24 L26
  constraint coincident L24 L27.end
  constraint perpendicular L24 L27
  constraint coincident L24 L28.end
  constraint perpendicular L24 L28
  measures "d163" radius of A1
  measures "d164" radius of A2
  measures "d167" distance of L22 L23
  measures "d169" distance of L23 L25
  measures "d170" distance of L6 L22
  measures "d171" distance of L25 L26
  measures "d172" distance of L26 L27
  measures "d173" distance of L27 L28
extrude "Extrude20" cut sketch "Sketch26" sketch "Sketch26" against normal blind 0.001 contours L11 L12 L13 L14 L15 S0 S1 S2 S3 A1 A2 S4 of sketch 2 text T0 T1 T2 T3 T4 T5 bodies 1
ref_plane "WorkPlane5" through (13, 1.75, -16.75) normal (0, 1, 0) x (1, 0, 0)
sketch "Sketch28" plane through (13, 1.75, -16.75) normal (0, 1, 0) x (1, 0, 0)
  line L0 (-8.5, 2.55) -> (-10.5, 2.55)
  line L1 (-10.5, 2.55) -> (-10.5, -1.45)
  line L2 (-10.5, -1.45) -> (-8.5, -1.45)
  line L3 (-8.5, -1.45) -> (-8.5, 2.55)
  line L4 (13, 16.75) -> (-13, 16.75)
  line L5 (8, 6.75) -> (-7.1, 6.75)
  line L6 (-13, 16.75) -> (-13, -16.75)
  dimension "d180" = 2
  dimension "d181" = 4
  dimension "d182" = 14.2
  dimension "d183" = 4.2
  dimension "d184" = 2.5
  constraint horizontal L0
  constraint vertical L1
  constraint horizontal L2
  constraint vertical L3
  measures "d180" distance of L0.start L0.end
  measures "d181" distance of L0.start L2.end
  measures "d182" distance of L0 L4
  measures "d183" distance of L0 L5
  measures "d184" distance of L1 L6
ref_plane "WorkPlane6" through (4, 2.75, -17.3) normal (-1, 0, 0) x (0, 0, 1)
sketch "Sketch29" plane through (4, 2.75, -17.3) normal (-1, 0, 0) x (0, 0, -1)
  line L0 (2.1, 1.2) -> (2.1, 0)
  line L1 (0, -1) -> (0, 1) construction
  line L2 (2, -1) -> (-2, -1) construction
  line L3 (2, 1) -> (-2, 1) construction
  line L4 (2.1, 0) -> (2, 0)
  line L5 (2, 1) -> (2, -1)
  line L6 (2.2, 1.2) -> (2.2, 0)
  line L7 (2.1, -0.1) -> (2, -0.1)
  arc A0 (2.1, -0.1) -> (2.2, 0) centre (2.1, 0) ccw
  line L8 (-2.2, 1.2) -> (-2.2, 0)
  arc A1 (-2.2, 0) -> (-2.1, -0.1) centre (-2.1, 0) ccw
  line L9 (-2.1, 0) -> (-2, 0)
  line L10 (-2.1, 1.2) -> (-2.1, 0)
  line L11 (-2.1, -0.1) -> (-2, -0.1)
  line L12 (16.2, 1.2) -> (-17.3, 1.2)
  line L13 (2.2, 1.2) -> (2.1, 1.2)
  line L14 (-2.1, 1.2) -> (-2.2, 1.2)
  line L15 (-2, -0.1) -> (-2, 0)
  line L16 (2, -0.1) -> (2, 0)
  dimension "d188" = 0.1
  dimension "d190" = 0.1
  dimension "d191" = 0.1
  dimension "d192" = 0.1
  constraint vertical L0
  constraint vertical L1
  constraint midpoint L1.start L2
  constraint midpoint L1.end L3
  constraint perpendicular L0 L4
  constraint midpoint L4.end L5
  constraint parallel L0 L6
  constraint parallel L4 L7
  constraint tangent L6 A0
  constraint tangent L7 A0
  constraint symmetric L0.start L1 L10.start
  constraint symmetric L0.end L1 A1.centre
  constraint symmetric L1 L4.end L9.end
  constraint symmetric L1 L6.start L8.start
  constraint symmetric L1 L7.end L11.end
  constraint symmetric L1 L6.end L8.end
  constraint symmetric L1 L7.start A1.end
  constraint symmetric L1 A0 A1
  constraint coincident L6.start L12
  constraint coincident L0.start L12
  constraint coincident L5 L7.end
  measures "d188" distance of L0.end L4.end
  measures "d190" radius of A0
  measures "d191" distance of L0 L6
  measures "d192" distance of L4 L7
sketch "Sketch30" plane through (0, 1.55, 0) normal (0, 1, 0) x (-1, 0, 0)
  circle A0 centre (-8.4, -28.1) radius 0.5
  circle A1 centre (-13.4, -28.1) radius 0.5
  circle A2 centre (-18.4, -28.1) radius 0.5
  line L0 (-19.48, -2.52) -> (-19.98, -2.52)
  line L1 (-19.98, -2.52) -> (-19.98, -2.02)
  line L2 (-19.98, -2.02) -> (-19.48, -2.02)
  line L3 (-19.48, -2.02) -> (-19.48, -2.52)
  line L4 (-16.94, -2.52) -> (-17.44, -2.52)
  line L5 (-17.44, -2.52) -> (-17.44, -2.02)
  line L6 (-17.44, -2.02) -> (-16.94, -2.02)
  line L7 (-16.94, -2.02) -> (-16.94, -2.52)
  line L8 (-14.4, -2.52) -> (-14.9, -2.52)
  line L9 (-14.9, -2.52) -> (-14.9, -2.02)
  line L10 (-14.9, -2.02) -> (-14.4, -2.02)
  line L11 (-14.4, -2.02) -> (-14.4, -2.52)
  circle A3 centre (-2.275, -2.375) radius 1.475
  circle A4 centre (-23.725, -2.375) radius 1.475
  circle A5 centre (-23.725, -31.325) radius 1.475
  circle A6 centre (-2.275, -31.325) radius 1.475
  line L12 (0, -33.5) -> (0, 0)
  line L13 (0, 0) -> (-26, 0)
  line L14 (-26, 0) -> (-26, -33.5)
  line L15 (-26, -33.5) -> (0, -33.5)
  line L16 (-4.5, -11.8) -> (-2.5, -11.8)
  line L17 (-2.5, -11.8) -> (-2.5, -10.8)
  line L18 (-2.5, -10.8) -> (-4.5, -10.8)
  line L19 (-4.5, -10.8) -> (-4.5, -11.8)
  line L20 (-4.5, -15.3) -> (-4.5, -19.3)
  line L21 (-2.5, -15.3) -> (-4.5, -15.3)
  dimension "d195" = 2
  dimension "d196" = 1
  dimension "d197" = 3.5
  constraint horizontal L16
  constraint vertical L17
  constraint horizontal L18
  constraint vertical L19
  constraint collinear L19 L20
  measures "d195" distance of L16.start L16.end
  measures "d196" distance of L16.start L18.end
  measures "d197" distance of L16 L21
sketch "Sketch31" plane through (0, 1.55, 0) normal (0, 1, 0) x (-1, 0, 0)
  circle A0 centre (-8.4, -28.1) radius 0.5
  circle A1 centre (-13.4, -28.1) radius 0.5
  circle A2 centre (-18.4, -28.1) radius 0.5
  line L0 (-19.48, -2.52) -> (-19.98, -2.52)
  line L1 (-19.98, -2.52) -> (-19.98, -2.02)
  line L2 (-19.98, -2.02) -> (-19.48, -2.02)
  line L3 (-19.48, -2.02) -> (-19.48, -2.52)
  line L4 (-16.94, -2.52) -> (-17.44, -2.52)
  line L5 (-17.44, -2.52) -> (-17.44, -2.02)
  line L6 (-17.44, -2.02) -> (-16.94, -2.02)
  line L7 (-16.94, -2.02) -> (-16.94, -2.52)
  line L8 (-14.4, -2.52) -> (-14.9, -2.52)
  line L9 (-14.9, -2.52) -> (-14.9, -2.02)
  line L10 (-14.9, -2.02) -> (-14.4, -2.02)
  line L11 (-14.4, -2.02) -> (-14.4, -2.52)
  circle A3 centre (-2.275, -2.375) radius 1.475
  circle A4 centre (-23.725, -2.375) radius 1.475
  circle A5 centre (-23.725, -31.325) radius 1.475
  circle A6 centre (-2.275, -31.325) radius 1.475
  line L12 (0, -33.5) -> (0, 0)
  line L13 (0, 0) -> (-26, 0)
  line L14 (-26, 0) -> (-26, -33.5)
  line L15 (-26, -33.5) -> (0, -33.5)
  line L16 (-3.75, -11.8) -> (-3.25, -11.8)
  line L17 (-3.25, -11.8) -> (-3.25, -12.3)
  line L18 (-3.25, -12.3) -> (-3.75, -12.3)
  line L19 (-3.75, -12.3) -> (-3.75, -11.8)
  line L20 (-3.5, -12.3) -> (-3.5, -10.8) construction
  line L21 (-2.5, -10.8) -> (-4.5, -10.8) construction
  line L22 (-4.5, -11.8) -> (-2.5, -11.8) construction
  line L23 (-4.5, -10.8) -> (-4, -10.8)
  line L24 (-4, -10.8) -> (-4, -10.3)
  line L25 (-4, -10.3) -> (-4.5, -10.3)
  line L26 (-4.5, -10.3) -> (-4.5, -10.8)
  line L27 (-3, -10.8) -> (-3, -10.3)
  line L28 (-2.5, -10.3) -> (-2.5, -10.8)
  line L29 (-3, -10.3) -> (-2.5, -10.3)
  line L30 (-2.5, -10.8) -> (-3, -10.8)
  point P0 (-2.5, -10.8)
  dimension "d200" = 0.5
  dimension "d201" = 0.5
  dimension "d202" = 0.5
  dimension "d203" = 0.5
  constraint horizontal L16
  constraint vertical L17
  constraint horizontal L18
  constraint vertical L19
  constraint midpoint L18 L20.start
  constraint perpendicular L18 L20
  constraint midpoint L20.end L21
  constraint collinear L16 L22
  constraint horizontal L23
  constraint vertical L24
  constraint horizontal L25
  constraint vertical L26
  constraint coincident L21.end L23.start
  constraint symmetric L20 L21.end P0
  constraint symmetric L20 L23.end L27.start
  constraint symmetric L20 L24.end L27.end
  constraint symmetric L20 L25.end L28.start
  measures "d200" distance of L17 L19
  measures "d201" distance of L16.start L18.end
  measures "d202" distance of L21.end L23.end
  measures "d203" distance of L21.end L25.end
sketch "Sketch32" plane through (0, 1.55, 0) normal (0, 1, 0) x (-1, 0, 0)
  circle A0 centre (-8.4, -28.1) radius 0.5
  circle A1 centre (-13.4, -28.1) radius 0.5
  circle A2 centre (-18.4, -28.1) radius 0.5
  line L0 (-19.48, -2.52) -> (-19.98, -2.52)
  line L1 (-19.98, -2.52) -> (-19.98, -2.02)
  line L2 (-19.98, -2.02) -> (-19.48, -2.02)
  line L3 (-19.48, -2.02) -> (-19.48, -2.52)
  line L4 (-16.94, -2.52) -> (-17.44, -2.52)
  line L5 (-17.44, -2.52) -> (-17.44, -2.02)
  line L6 (-17.44, -2.02) -> (-16.94, -2.02)
  line L7 (-16.94, -2.02) -> (-16.94, -2.52)
  line L8 (-14.4, -2.52) -> (-14.9, -2.52)
  line L9 (-14.9, -2.52) -> (-14.9, -2.02)
  line L10 (-14.9, -2.02) -> (-14.4, -2.02)
  line L11 (-14.4, -2.02) -> (-14.4, -2.52)
  circle A3 centre (-2.275, -2.375) radius 1.475
  circle A4 centre (-23.725, -2.375) radius 1.475
  circle A5 centre (-23.725, -31.325) radius 1.475
  circle A6 centre (-2.275, -31.325) radius 1.475
  line L12 (0, -33.5) -> (0, 0)
  line L13 (0, 0) -> (-26, 0)
  line L14 (-26, 0) -> (-26, -33.5)
  line L15 (-26, -33.5) -> (0, -33.5)
  line L16 (-2.3, -9) -> (-3.3, -9)
  line L17 (-3.3, -9) -> (-3.3, -7.5)
  line L18 (-3.3, -7.5) -> (-2.3, -7.5)
  line L19 (-2.3, -7.5) -> (-2.3, -9)
  line L20 (-2.5, -11.8) -> (-2.5, -10.8)
  line L21 (-2.5, -10.8) -> (-4.5, -10.8)
  dimension "d206" = 1
  dimension "d207" = 1.5
  dimension "d208" = 0.2
  dimension "d209" = 1.8
  constraint horizontal L16
  constraint vertical L17
  constraint horizontal L18
  constraint vertical L19
  measures "d206" distance of L16.start L16.end
  measures "d207" distance of L16.start L18.end
  measures "d208" distance of L19 L20
  measures "d209" distance of L16 L21
sketch "Sketch33" plane through (2.3, 0, 0) normal (-1, 0, 0) x (0, 0, 1)
  line L0 (-9, 1.55) -> (-7.5, 1.55)
  line L1 (-7.5, 1.55) -> (-7.5, 1.8)
  line L2 (-7.5, 1.8) -> (-9, 1.8)
  line L3 (-9, 1.8) -> (-9, 1.55)
  line L4 (-7.5, 1.55) -> (-7.5, 1.6)
  line L5 (-7.5, 1.55) -> (-7.45, 1.55)
  arc A0 (-7.45, 1.55) -> (-7.5, 1.6) centre (-7.5, 1.55) ccw
  line L6 (-8.25, 1.8) -> (-8.25, 1.55) construction
  line L7 (-9, 1.55) -> (-9, 1.6)
  arc A1 (-9, 1.6) -> (-9.05, 1.55) centre (-9, 1.55) ccw
  line L8 (-9, 1.55) -> (-9.05, 1.55)
  dimension "d212" = 0.1
  constraint coincident L0.end L1.start
  constraint coincident L1 L4.end
  constraint perpendicular L0 L4
  constraint perpendicular L4 L5
  constraint midpoint L2 L6.start
  constraint midpoint L0 L6.end
  constraint symmetric L0.end L6 L0.start
  constraint symmetric L4.end L6 L7.end
  constraint symmetric L5.end L6 A1.end
  constraint symmetric A0 L6 A1
  measures "d212" diameter of A0
sketch "Sketch34" plane through (0, 1.8, 0) normal (0, 1, 0) x (-1, 0, 0)
  line L0 (-2.3, -7.5) -> (-3.3, -7.5)
  line L1 (-3.3, -7.5) -> (-3.3, -9)
  line L2 (-3.3, -9) -> (-2.3, -9)
  line L3 (-2.3, -9) -> (-2.3, -7.5)
  line L4 (-3.0427, -7.5) -> (-3.0427, -9) construction
  constraint coincident L0 L4.start
  constraint coincident L2 L4.end
  constraint perpendicular L2 L4
sketch "Sketch35" plane through (0, 1.55, 0) normal (0, 1, 0) x (-1, 0, 0)
  circle A0 centre (-8.4, -28.1) radius 0.5
  circle A1 centre (-13.4, -28.1) radius 0.5
  circle A2 centre (-18.4, -28.1) radius 0.5
  line L0 (-19.48, -2.52) -> (-19.98, -2.52)
  line L1 (-19.98, -2.52) -> (-19.98, -2.02)
  line L2 (-19.98, -2.02) -> (-19.48, -2.02)
  line L3 (-19.48, -2.02) -> (-19.48, -2.52)
  line L4 (-16.94, -2.52) -> (-17.44, -2.52)
  line L5 (-17.44, -2.52) -> (-17.44, -2.02)
  line L6 (-17.44, -2.02) -> (-16.94, -2.02)
  line L7 (-16.94, -2.02) -> (-16.94, -2.52)
  line L8 (-14.4, -2.52) -> (-14.9, -2.52)
  line L9 (-14.9, -2.52) -> (-14.9, -2.02)
  line L10 (-14.9, -2.02) -> (-14.4, -2.02)
  line L11 (-14.4, -2.02) -> (-14.4, -2.52)
  circle A3 centre (-2.275, -2.375) radius 1.475
  circle A4 centre (-23.725, -2.375) radius 1.475
  circle A5 centre (-23.725, -31.325) radius 1.475
  circle A6 centre (-2.275, -31.325) radius 1.475
  line L12 (0, -33.5) -> (0, 0)
  line L13 (0, 0) -> (-26, 0)
  line L14 (-26, 0) -> (-26, -33.5)
  line L15 (-26, -33.5) -> (0, -33.5)
  line L16 (-7.8, -2.5) -> (-10.3, -2.5)
  line L17 (-10.3, -2.5) -> (-10.3, -1.5)
  line L18 (-10.3, -1.5) -> (-7.8, -1.5)
  line L19 (-7.8, -1.5) -> (-7.8, -2.5)
  line L20 (-13.38, -3.032) -> (-13.38, -1.508)
  dimension "d217" = 2.5
  dimension "d218" = 1
  dimension "d219" = 7.8
  dimension "d220" = 3.88
  dimension "d221" = 1.5
  constraint horizontal L16
  constraint vertical L17
  constraint horizontal L18
  constraint vertical L19
  measures "d217" distance of L16.start L16.end
  measures "d218" distance of L16.start L18.end
  measures "d219" distance of L12 L19
  measures "d221" distance of L13 L18
sketch "Sketch36" plane through (7.8, 0, 0) normal (-1, 0, 0) x (0, 0, 1)
  line L0 (-2.5, 1.55) -> (-1.5, 1.55)
  line L1 (-1.5, 1.55) -> (-1.5, 2.05)
  line L2 (-1.5, 2.05) -> (-2.5, 2.05)
  line L3 (-2.5, 2.05) -> (-2.5, 1.55)
sketch "Sketch37" plane through (10.3, 0, 0) normal (1, 0, 0) x (0, 0, -1)
  line L0 (1.5, 1.55) -> (2.5, 1.55)
  line L1 (2.5, 1.55) -> (2.5, 2.05)
  line L2 (2.5, 2.05) -> (1.5, 2.05)
  line L3 (1.5, 2.05) -> (1.5, 1.55)